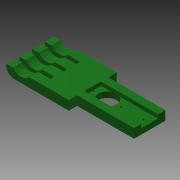
# Autodesk Inventor part: hand1
Saved by Autodesk Inventor 2013 (Build 170138000, 138)
## iProperties
Created: 2014-06-28
Part Number: hand1
Material: Generic
Document SubType Name: Modeling
Designer: Masta
Density: 1 g/cm^3
Author: Masta
Autodesk Inventor part; units mm, degrees
ref_plane "YZ Plane" through (0, 0, 0) normal (1, 0, 0) x (0, 1, 0)
ref_plane "XZ Plane" through (0, 0, 0) normal (0, 1, 0) x (-1, 0, 0)
ref_plane "XY Plane" through (0, 0, 0) normal (0, 0, 1) x (1, 0, 0)
sketch "Sketch1" plane through (0, 0, 0) normal (0, 0, 1) x (1, 0, 0)
  arc A0 (2.1794, -4.5) -> (2.1794, 4.5) centre (0, 0) ccw
  line L0 (-23, -4.5) -> (-2.1794, -4.5)
  line L1 (23, -4.5) -> (23, 4.5)
  line L2 (23, 4.5) -> (2.1794, 4.5)
  line L3 (-23, 4.5) -> (-23, -4.5)
  line L4 (-23, -4.5) -> (23, 4.5) construction
  line L5 (23, -4.5) -> (-23, 4.5) construction
  line L6 (0, 0) -> (23, 0) construction
  line L7 (0, 0) -> (0, 4.5) construction
  line L8 (23, -8.5) -> (-23, -8.5)
  line L9 (-23, -8.5) -> (-23, 8.5)
  line L10 (-23, 8.5) -> (23, 8.5)
  line L11 (23, 8.5) -> (23, -8.5)
  line L12 (23, -8.5) -> (-23, 8.5) construction
  line L13 (-23, -8.5) -> (23, 8.5) construction
  line L14 (-2.1794, 4.5) -> (-23, 4.5)
  line L15 (2.1794, 4.5) -> (-2.1794, 4.5)
  line L16 (-2.1794, -4.5) -> (2.1794, -4.5)
  line L17 (2.1794, -4.5) -> (23, -4.5)
  arc A1 (-2.1794, -4.5) -> (2.1794, -4.5) centre (0, 0) ccw
  arc A2 (2.1794, 4.5) -> (-2.1794, 4.5) centre (0, 0) ccw
  arc A3 (-2.1794, 4.5) -> (-2.1794, -4.5) centre (0, 0) ccw
  point P0 (7.62, 0)
  point P1 (19.62, 0)
  point P2 (-7.62, 0)
  point P3 (-19.62, 0)
  point P4 (20, 0)
  dimension "d0" = 10
  dimension "d1" = 46
  dimension "d2" = 9
  dimension "d3" = 7.62
  dimension "d4" = 12
  dimension "d5" = 4
  constraints: 36 end point, 12 parallel, 9 point on circle, 6 midpoint, 4 centre point, 4 horizontal, 4 perpendicular, 3 point on line, 2 symmetric about line, 1 coincident, 1 collinear
  measures "d0" diameter of A0
  measures "d1" distance of L3.start L1.end
  measures "d2" distance of L1.end L1.start
  measures "d3" distance of L6.start point (7.62, 0)
  measures "d4" distance of point (19.62, 0) point (7.62, 0)
  measures "d5" distance between parallel lines of L10 L2
extrude "Extrusion1" add sketch "Sketch1" against normal blind 3 contours A0 L2 L1 L17 | L17 L11 L8 L9 L0 A1 | A2 L14 L9 L10 L11 L2 | L0 L3 L14 A3
extrude "Extrusion2" add sketch "Sketch1" along normal blind 2 contours A1 L16 | L17 L11 L8 L9 L0 A1 | A2 L14 L9 L10 L11 L2 | L15 A2
sketch "Sketch2" plane through (0, 0, -3) normal (0, 0, -1) x (-1, 0, 0)
  circle A0 centre (0, 0) radius 5 projected
  line L0 (8, 6) -> (42, 6)
  line L1 (42, 6) -> (42, 1)
  line L2 (42, 1) -> (8, 1)
  line L3 (8, 1) -> (8, 6)
  line L4 (-23, -8.5) -> (23, -8.5) projected
  line L5 (23, 8.5) -> (-23, 8.5) projected
  line L6 (-23, 8.5) -> (-23, -8.5) projected
  line L7 (8, 8.5) -> (8, -8.5)
  line L8 (23, -8.5) -> (23, 8.5) projected
  line L9 (8, -8.5) -> (23, -8.5)
  line L10 (23, 8.5) -> (23, -8.5)
  line L11 (23, 8.5) -> (8, 8.5)
  dimension "d12" = 8
  dimension "d13" = 34
  dimension "d14" = 5
  dimension "d15" = 1
  constraints: 16 end point, 4 collinear, 3 parallel, 2 point on line, 1 horizontal, 1 perpendicular
  measures "d12" distance from line of L3 A0.centre
  measures "d13" distance of L0.start L0.end
  measures "d14" distance of L0.end L1.end
  measures "d15" distance from line of L2 A0.centre
extrude "Extrusion3" add sketch "Sketch2" against normal up to surface (5 mm away) contours L0 L8 L2 L3 | L0 L1 L2 L8
sketch "Sketch3" plane through (-42, 6, -3) normal (0, 1, 0) x (1, 0, 0)
  line L0 (0, -5) -> (19, -5) projected
  arc A0 (12.5, -5) -> (3.5, -5) centre (8, -8.9686) ccw
  point P0 (42, -3)
  dimension "d33" = 6
  dimension "d35" = 3.5
  dimension "d36" = 9
  constraints: 2 point on circle, 2 point on line, 1 centre point
  measures "d33" radius of A0
  measures "d35" distance of L0.start A0.end
  measures "d36" distance of A0.start A0.end
extrude "Extrusion4" cut sketch "Sketch3" against normal up to next
pattern_linear "Rectangular Pattern1" count 4 spacing 7 along (0, -1, 0) of "Extrusion3", "Extrusion4" first direction both ways yes
extrude "Extrusion5" add sketch "Sketch2" against normal up to surface (5 mm away) contours L7 L5 L8 L0 | L0 L8 L2 L3 | L2 L8 L4 L7
hole "Hole1" at (7.62, 0, 0) at (19.62, 0, 0) at (-19.62, 0, 0) at (-7.62, 0, 0) direction (0, 0, -1) diameter 1 end through all
fillet "Fillet1" radius 4 3 edges at (-42, -10.5, -3) (-42, 3.5, -3) (-42, -3.5, -3)
body "Solid1"
